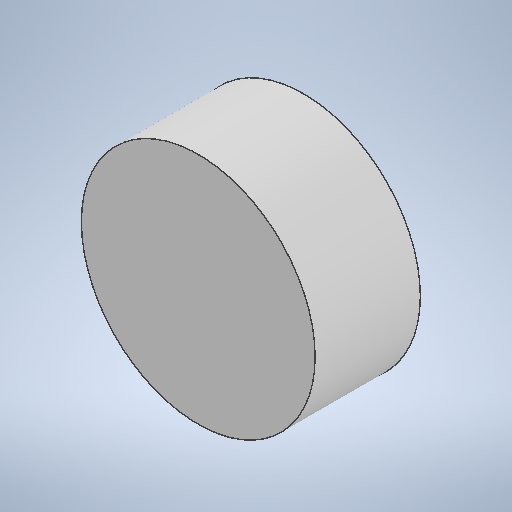
# Autodesk Inventor part: wheel
Saved by Autodesk Inventor 2025 (Build 290162000, 162)
## iProperties
Created: 2025-10-18
Part Number: wheel
Material: 一般
Document SubType Name: Modeling
Designer: sooo1
Density: 1 g/cm^3
Appearance: 既定
Author: sooo1
Autodesk Inventor part; units mm, degrees
ref_plane "YZ Plane" through (0, 0, 0) normal (1, 0, 0) x (0, 1, 0)
ref_plane "XZ Plane" through (0, 0, 0) normal (0, 1, 0) x (-1, 0, 0)
ref_plane "XY Plane" through (0, 0, 0) normal (0, 0, 1) x (1, 0, 0)
sketch "スケッチ1" plane through (0, 0, 0) normal (0, 0, 1) x (1, 0, 0)
  circle A0 centre (0, 0) radius 10
  circle A1 centre (0, 0) radius 9
  line L0 (-14, 0) -> (14, 0) construction
  line L1 (0, -14) -> (0, 14) construction
  circle A2 centre (-6, 0) radius 2.05
  circle A3 centre (6, 0) radius 2.05
  dimension "d0" = 20
  dimension "d1" = 18
  dimension "d2" = 4.1
  dimension "d3" = 6
  constraints: 4 centre point, 2 coincident, 1 point on line, 1 symmetric about line, 1 other
  measures "d0" diameter of A0
  measures "d1" diameter of A1
  measures "d2" diameter of A2
  measures "d3" distance from line of L1 A2.centre
extrude "押し出し1" add sketch "スケッチ1" along normal blind 9 contours A0 | A1 | A2 | A3
extrude "押し出し2" cut sketch "スケッチ1" along normal blind 2 contours A1
extrude "押し出し4" add sketch "スケッチ1" against normal blind 0.88 contours A2 | A3
chamfer "面取り1" distance 0.3 angle 45 2 edges at (-8.05, 0, -0.88) (3.95, 0, -0.88)
